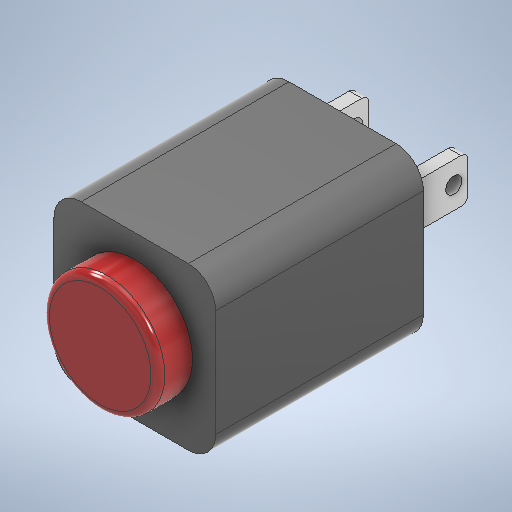
# Autodesk Inventor part: PWR BTN
Saved by Autodesk Inventor 2025 (Build 290162000, 162)
## iProperties
Created: 2025-05-10
Part Number: PWR BTN
Material: Generic
Document SubType Name: Modeling
Designer: thesn
Density: 1 g/cm^3
Appearance: Default
Author: thesn
Autodesk Inventor part; units mm, degrees
ref_plane "YZ Plane" through (0, 0, 0) normal (1, 0, 0) x (0, 1, 0)
ref_plane "XZ Plane" through (0, 0, 0) normal (0, 1, 0) x (-1, 0, 0)
ref_plane "XY Plane" through (0, 0, 0) normal (0, 0, 1) x (1, 0, 0)
sketch "Sketch1" plane through (0, 0, 0) normal (0, 0, 1) x (1, 0, 0)
  line L0 (0, 0) -> (17.78, 0)
  line L1 (17.78, 0) -> (17.78, 17.78)
  line L2 (17.78, 17.78) -> (0, 17.78)
  line L3 (0, 17.78) -> (0, 0)
  dimension "d0" = 17.78
  dimension "d1" = 17.78
  constraints: 8 end point, 2 parallel, 1 horizontal, 1 perpendicular
  measures "d0" distance of L2.end L1.end
  measures "d1" distance of L1.end L0.end
extrude "Extrusion1" add sketch "Sketch1" against normal blind 22.86
fillet "Fillet1" radius 3 4 edges at (17.78, 17.78, -11.43) (0, 17.78, -11.43) (17.78, 0, -11.43) (0, 0, -11.43)
sketch "Sketch2" plane through (0, 0, 0) normal (0, 0, 1) x (1, 0, 0)
  circle A0 centre (8.89, 8.89) radius 6.35
  line L0 (14.78, 17.78) -> (3, 17.78) projected
  line L1 (0, 14.78) -> (0, 3) projected
  point P0 (0, 0)
  point P1 (8.89, 17.78)
  point P2 (0, 8.89)
  dimension "d5" = 0
  dimension "d6" = 0
  dimension "d7" = 12.7
  constraints: 2 midpoint, 1 centre point
  measures "d5" horizontal distance of point (8.89, 17.78) A0.centre
  measures "d6" vertical distance of point (0, 8.89) A0.centre
  measures "d7" diameter of A0
extrude "Extrusion2" add sketch "Sketch2" along normal blind 3.81
fillet "Fillet2" radius 0.762 1 edges at (2.54, 8.89, 3.81)
sketch "Sketch3" plane through (0, 0, -22.86) normal (0, 0, -1) x (-1, 0, 0)
  line L0 (-15.0625, 13.3567) -> (-13.6709, 13.3567)
  line L1 (-13.6709, 13.3567) -> (-13.6709, 8.5084)
  line L2 (-13.6709, 8.5084) -> (-15.0625, 8.5084)
  line L3 (-15.0625, 8.5084) -> (-15.0625, 13.3567)
  line L4 (-4.1566, 13.3567) -> (-2.7649, 13.3567)
  line L5 (-2.7649, 13.3567) -> (-2.7649, 8.5084)
  line L6 (-2.7649, 8.5084) -> (-4.1566, 8.5084)
  line L7 (-4.1566, 8.5084) -> (-4.1566, 13.3567)
  line L8 (-3, 17.78) -> (-14.78, 17.78) projected
  point P0 (0, 0)
  point P1 (-3.4608, 13.3567)
  point P2 (-14.3667, 13.3567)
  point P3 (-8.89, 17.78)
  dimension "d11" = 0
  dimension "d12" = 5.4767
  dimension "d13" = 1.3916
  dimension "d14" = 4.8482
  dimension "d15" = 4.8482
  dimension "d16" = 1.3916
  constraints: 16 end point, 4 parallel, 3 midpoint, 2 horizontal, 2 perpendicular
  measures "d11" vertical distance of point (-3.461, 13.357) point (-14.367, 13.357)
  measures "d12" horizontal distance of point (-8.89, 17.78) point (-14.367, 13.357)
  measures "d13" distance between parallel lines of L1 L3
  measures "d14" distance between parallel lines of L2 L0
  measures "d15" distance between parallel lines of L6 L4
  measures "d16" distance between parallel lines of L7 L5
extrude "Extrusion3" add sketch "Sketch3" along normal blind 7.62
sketch "Sketch4" plane through (2.7649, 8.5084, -22.86) normal (-1, 0, 0) x (0, 0, 1)
  circle A0 centre (-6.0701, 2.4241) radius 0.889
  point P0 (22.86, -8.5084)
  dimension "d19" = 1.778
  constraints: 1 centre point
  measures "d19" diameter of A0
extrude "Extrusion4" cut sketch "Sketch4" against normal blind 25.4
fillet "Fillet3" radius 0.762 4 edges at (14.3667, 13.3567, -30.48) (3.4608, 13.3567, -30.48) (14.3667, 8.5084, -30.48) (3.4608, 8.5084, -30.48)
sketch "Sketch5" plane through (0, 0, -22.86) normal (0, 0, -1) x (-1, 0, 0)
  line L0 (-16.1365, 4.1263) -> (18.4067, 4.1263) construction
  line L1 (18.4067, 4.1263) -> (18.4067, 0.8585) construction
  line L2 (18.4067, 0.8585) -> (-16.1365, 0.8585) construction
  line L3 (-16.1365, 0.8585) -> (-16.1365, 4.1263) construction
  line L4 (-16.1448, 2.7914) -> (-15.7166, 4.0614)
  line L5 (-15.7166, 4.0614) -> (-15.5087, 4.0614)
  line L6 (-15.5087, 4.0614) -> (-15.0806, 2.7914)
  line L7 (-15.0806, 2.7914) -> (-15.2586, 2.7914)
  line L8 (-15.2586, 2.7914) -> (-15.3739, 3.1465)
  line L9 (-15.3739, 3.1465) -> (-15.8586, 3.1465)
  line L10 (-15.8586, 3.1465) -> (-15.9739, 2.7914)
  line L11 (-15.9739, 2.7914) -> (-16.1448, 2.7914)
  line L12 (-15.4202, 3.2906) -> (-15.6168, 3.8885)
  line L13 (-15.6168, 3.8885) -> (-15.8123, 3.2906)
  line L14 (-15.8123, 3.2906) -> (-15.4202, 3.2906)
  line L15 (-14.2398, 2.7914) -> (-14.4003, 2.7914)
  line L16 (-14.4003, 2.7914) -> (-14.4003, 2.8882)
  spline S0 degree 2 poles (-14.4003, 2.8882) (-14.4374, 2.8573) (-14.4919, 2.8161) (-14.5289, 2.7987) knots 0 0 0 1 2 2 2
  spline S1 degree 2 poles (-14.5289, 2.7987) (-14.5629, 2.7822) (-14.636, 2.7647) (-14.6844, 2.7647) knots 0 0 0 1 2 2 2
  spline S2 degree 2 poles (-14.6844, 2.7647) (-14.7626, 2.7647) (-14.8943, 2.8295) (-14.9406, 2.8923) knots 0 0 0 1 2 2 2
  spline S3 degree 2 poles (-14.9406, 2.8923) (-14.9869, 2.9551) (-15.0384, 3.1403) (-15.0384, 3.2608) knots 0 0 0 1 2 2 2
  spline S4 degree 2 poles (-15.0384, 3.2608) (-15.0384, 3.3863) (-14.9736, 3.5695) (-14.9169, 3.6385) knots 0 0 0 1 2 2 2
  spline S5 degree 2 poles (-14.9169, 3.6385) (-14.8645, 3.7002) (-14.7173, 3.7712) (-14.636, 3.7712) knots 0 0 0 1 2 2 2
  spline S6 degree 2 poles (-14.636, 3.7712) (-14.565, 3.7712) (-14.459, 3.7393) (-14.4003, 3.7064) knots 0 0 0 1 2 2 2
  line L17 (-14.4003, 3.7064) -> (-14.4003, 4.1181)
  line L18 (-14.4003, 4.1181) -> (-14.2398, 4.1181)
  line L19 (-14.2398, 4.1181) -> (-14.2398, 2.7914)
  line L20 (-14.4003, 3.023) -> (-14.4003, 3.5736)
  spline S7 degree 2 poles (-14.4003, 3.5736) (-14.46, 3.6024) (-14.5547, 3.6241) (-14.6092, 3.6241) knots 0 0 0 1 2 2 2
  spline S8 degree 2 poles (-14.6092, 3.6241) (-14.7327, 3.6241) (-14.8727, 3.4388) (-14.8727, 3.2638) knots 0 0 0 1 2 2 2
  spline S9 degree 2 poles (-14.8727, 3.2638) (-14.8727, 3.0951) (-14.7657, 2.917) (-14.6473, 2.917) knots 0 0 0 1 2 2 2
  spline S10 degree 2 poles (-14.6473, 2.917) (-14.5845, 2.917) (-14.4569, 2.9746) (-14.4003, 3.023) knots 0 0 0 1 2 2 2
  spline S11 degree 2 poles (-13.4761, 2.8923) (-13.4957, 2.8779) (-13.5615, 2.8264) (-13.5924, 2.811) knots 0 0 0 1 2 2 2
  spline S12 degree 2 poles (-13.5924, 2.811) (-13.6346, 2.7884) (-13.7138, 2.7647) (-13.7859, 2.7647) knots 0 0 0 1 2 2 2
  spline S13 degree 2 poles (-13.7859, 2.7647) (-13.8445, 2.7647) (-13.9506, 2.8089) (-13.9907, 2.8491) knots 0 0 0 1 2 2 2
  spline S14 degree 2 poles (-13.9907, 2.8491) (-14.0288, 2.8882) (-14.0751, 3.0035) (-14.0751, 3.0673) knots 0 0 0 1 2 2 2
  spline S15 degree 2 poles (-14.0751, 3.0673) (-14.0751, 3.1661) (-13.9917, 3.306) (-13.9012, 3.3462) knots 0 0 0 1 2 2 2
  spline S16 degree 2 poles (-13.9012, 3.3462) (-13.8209, 3.3832) (-13.6027, 3.411) (-13.4761, 3.4182) knots 0 0 0 1 2 2 2
  line L21 (-13.4761, 3.4182) -> (-13.4761, 3.4491)
  spline S17 degree 2 poles (-13.4761, 3.4491) (-13.4761, 3.5047) (-13.5101, 3.5736) (-13.5409, 3.5932) knots 0 0 0 1 2 2 2
  spline S18 degree 2 poles (-13.5409, 3.5932) (-13.5718, 3.6127) (-13.6603, 3.6251) (-13.7077, 3.6251) knots 0 0 0 1 2 2 2
  spline S19 degree 2 poles (-13.7077, 3.6251) (-13.7632, 3.6251) (-13.9135, 3.5921) (-13.9886, 3.5602) knots 0 0 0 1 2 2 2
  line L22 (-13.9886, 3.5602) -> (-13.9979, 3.5602)
  line L23 (-13.9979, 3.5602) -> (-13.9979, 3.7239)
  spline S20 degree 2 poles (-13.9979, 3.7239) (-13.9536, 3.7362) (-13.7879, 3.7671) (-13.7066, 3.7671) knots 0 0 0 1 2 2 2
  spline S21 degree 2 poles (-13.7066, 3.7671) (-13.6078, 3.7671) (-13.473, 3.7362) (-13.4195, 3.6961) knots 0 0 0 1 2 2 2
  spline S22 degree 2 poles (-13.4195, 3.6961) (-13.367, 3.657) (-13.3156, 3.5325) (-13.3156, 3.4429) knots 0 0 0 1 2 2 2
  line L24 (-13.3156, 3.4429) -> (-13.3156, 2.7914)
  line L25 (-13.3156, 2.7914) -> (-13.4761, 2.7914)
  line L26 (-13.4761, 2.7914) -> (-13.4761, 2.8923)
  line L27 (-13.4761, 3.0261) -> (-13.4761, 3.2906)
  spline S23 degree 2 poles (-13.4761, 3.2906) (-13.5337, 3.2855) (-13.7077, 3.268) (-13.7622, 3.2515) knots 0 0 0 1 2 2 2
  spline S24 degree 2 poles (-13.7622, 3.2515) (-13.826, 3.2319) (-13.9094, 3.1506) (-13.9094, 3.0786) knots 0 0 0 1 2 2 2
  spline S25 degree 2 poles (-13.9094, 3.0786) (-13.9094, 2.9963) (-13.8168, 2.9129) (-13.7283, 2.9129) knots 0 0 0 1 2 2 2
  spline S26 degree 2 poles (-13.7283, 2.9129) (-13.6531, 2.9129) (-13.5296, 2.9777) (-13.4761, 3.0261) knots 0 0 0 1 2 2 2
  line L28 (-12.589, 3.9637) -> (-12.5972, 3.9637)
  spline S27 degree 2 poles (-12.5972, 3.9637) (-12.6188, 3.9719) (-12.6991, 3.9863) (-12.731, 3.9863) knots 0 0 0 1 2 2 2
  spline S28 degree 2 poles (-12.731, 3.9863) (-12.8318, 3.9863) (-12.9183, 3.8958) (-12.9183, 3.7764) knots 0 0 0 1 2 2 2
  line L29 (-12.9183, 3.7764) -> (-12.9183, 3.7445)
  line L30 (-12.9183, 3.7445) -> (-12.6528, 3.7445)
  line L31 (-12.6528, 3.7445) -> (-12.6528, 3.6117)
  line L32 (-12.6528, 3.6117) -> (-12.9131, 3.6117)
  line L33 (-12.9131, 3.6117) -> (-12.9131, 2.7914)
  line L34 (-12.9131, 2.7914) -> (-13.0737, 2.7914)
  line L35 (-13.0737, 2.7914) -> (-13.0737, 3.6117)
  line L36 (-13.0737, 3.6117) -> (-13.1818, 3.6117)
  line L37 (-13.1818, 3.6117) -> (-13.1818, 3.7445)
  line L38 (-13.1818, 3.7445) -> (-13.0737, 3.7445)
  line L39 (-13.0737, 3.7445) -> (-13.0737, 3.7764)
  spline S29 degree 2 poles (-13.0737, 3.7764) (-13.0737, 3.9472) (-12.908, 4.1263) (-12.7536, 4.1263) knots 0 0 0 1 2 2 2
  spline S30 degree 2 poles (-12.7536, 4.1263) (-12.7094, 4.1263) (-12.6239, 4.117) (-12.589, 4.1108) knots 0 0 0 1 2 2 2
  line L40 (-12.589, 4.1108) -> (-12.589, 3.9637)
  line L41 (-12.0291, 3.5726) -> (-12.0373, 3.5726)
  spline S31 degree 2 poles (-12.0373, 3.5726) (-12.0558, 3.5777) (-12.096, 3.5798) (-12.1238, 3.5798) knots 0 0 0 1 2 2 2
  spline S32 degree 2 poles (-12.1238, 3.5798) (-12.1886, 3.5798) (-12.3162, 3.5232) (-12.3739, 3.4676) knots 0 0 0 1 2 2 2
  line L42 (-12.3739, 3.4676) -> (-12.3739, 2.7914)
  line L43 (-12.3739, 2.7914) -> (-12.5344, 2.7914)
  line L44 (-12.5344, 2.7914) -> (-12.5344, 3.7445)
  line L45 (-12.5344, 3.7445) -> (-12.3739, 3.7445)
  line L46 (-12.3739, 3.7445) -> (-12.3739, 3.6024)
  spline S33 degree 2 poles (-12.3739, 3.6024) (-12.2864, 3.6807) (-12.1557, 3.7445) (-12.0939, 3.7445) knots 0 0 0 1 2 2 2
  spline S34 degree 2 poles (-12.0939, 3.7445) (-12.0692, 3.7445) (-12.0445, 3.7424) (-12.0291, 3.7393) knots 0 0 0 1 2 2 2
  line L47 (-12.0291, 3.7393) -> (-12.0291, 3.5726)
  line L48 (-11.1636, 2.7914) -> (-11.3241, 2.7914)
  line L49 (-11.3241, 2.7914) -> (-11.3241, 2.8964)
  spline S35 degree 2 poles (-11.3241, 2.8964) (-11.3982, 2.8316) (-11.531, 2.7647) (-11.6133, 2.7647) knots 0 0 0 1 2 2 2
  spline S36 degree 2 poles (-11.6133, 2.7647) (-11.6751, 2.7647) (-11.7852, 2.8059) (-11.8253, 2.8501) knots 0 0 0 1 2 2 2
  spline S37 degree 2 poles (-11.8253, 2.8501) (-11.8665, 2.8944) (-11.9118, 3.0292) (-11.9118, 3.1259) knots 0 0 0 1 2 2 2
  line L50 (-11.9118, 3.1259) -> (-11.9118, 3.7445)
  line L51 (-11.9118, 3.7445) -> (-11.7512, 3.7445)
  line L52 (-11.7512, 3.7445) -> (-11.7512, 3.2011)
  spline S38 degree 2 poles (-11.7512, 3.2011) (-11.7512, 3.1249) (-11.7399, 3.0251) (-11.7203, 2.988) knots 0 0 0 1 2 2 2
  spline S39 degree 2 poles (-11.7203, 2.988) (-11.7008, 2.951) (-11.6339, 2.917) (-11.5711, 2.917) knots 0 0 0 1 2 2 2
  spline S40 degree 2 poles (-11.5711, 2.917) (-11.5124, 2.917) (-11.3797, 2.9839) (-11.3241, 3.0323) knots 0 0 0 1 2 2 2
  line L53 (-11.3241, 3.0323) -> (-11.3241, 3.7445)
  line L54 (-11.3241, 3.7445) -> (-11.1636, 3.7445)
  line L55 (-11.1636, 3.7445) -> (-11.1636, 2.7914)
  line L56 (-10.7673, 2.7914) -> (-10.9279, 2.7914)
  line L57 (-10.9279, 2.7914) -> (-10.9279, 3.7445)
  line L58 (-10.9279, 3.7445) -> (-10.7673, 3.7445)
  line L59 (-10.7673, 3.7445) -> (-10.7673, 2.7914)
  line L60 (-10.756, 3.903) -> (-10.9382, 3.903)
  line L61 (-10.9382, 3.903) -> (-10.9382, 4.0697)
  line L62 (-10.9382, 4.0697) -> (-10.756, 4.0697)
  line L63 (-10.756, 4.0697) -> (-10.756, 3.903)
  spline S41 degree 2 poles (-10.2435, 2.7729) (-10.3742, 2.7729) (-10.5213, 2.9222) (-10.5213, 3.0837) knots 0 0 0 1 2 2 2
  line L64 (-10.5213, 3.0837) -> (-10.5213, 3.6117)
  line L65 (-10.5213, 3.6117) -> (-10.6294, 3.6117)
  line L66 (-10.6294, 3.6117) -> (-10.6294, 3.7445)
  line L67 (-10.6294, 3.7445) -> (-10.5213, 3.7445)
  line L68 (-10.5213, 3.7445) -> (-10.5213, 4.0182)
  line L69 (-10.5213, 4.0182) -> (-10.3608, 4.0182)
  line L70 (-10.3608, 4.0182) -> (-10.3608, 3.7445)
  line L71 (-10.3608, 3.7445) -> (-10.0654, 3.7445)
  line L72 (-10.0654, 3.7445) -> (-10.0654, 3.6117)
  line L73 (-10.0654, 3.6117) -> (-10.3608, 3.6117)
  line L74 (-10.3608, 3.6117) -> (-10.3608, 3.1578)
  spline S42 degree 2 poles (-10.3608, 3.1578) (-10.3608, 3.0858) (-10.3557, 3.0065) (-10.3382, 2.9726) knots 0 0 0 1 2 2 2
  spline S43 degree 2 poles (-10.3382, 2.9726) (-10.3237, 2.9427) (-10.2589, 2.9129) (-10.2033, 2.9129) knots 0 0 0 1 2 2 2
  spline S44 degree 2 poles (-10.2033, 2.9129) (-10.1642, 2.9129) (-10.0912, 2.9366) (-10.0747, 2.9438) knots 0 0 0 1 2 2 2
  line L75 (-10.0747, 2.9438) -> (-10.0654, 2.9438)
  line L76 (-10.0654, 2.9438) -> (-10.0654, 2.7997)
  spline S45 degree 2 poles (-10.0654, 2.7997) (-10.1107, 2.7873) (-10.2033, 2.7729) (-10.2435, 2.7729) knots 0 0 0 1 2 2 2
  spline S46 degree 2 poles (-8.5865, 3.6786) (-8.5865, 3.5963) (-8.6452, 3.4481) (-8.6977, 3.3966) knots 0 0 0 1 2 2 2
  spline S47 degree 2 poles (-8.6977, 3.3966) (-8.7635, 3.3318) (-8.9416, 3.2649) (-9.0774, 3.2649) knots 0 0 0 1 2 2 2
  line L77 (-9.0774, 3.2649) -> (-9.2205, 3.2649)
  line L78 (-9.2205, 3.2649) -> (-9.2205, 2.7914)
  line L79 (-9.2205, 2.7914) -> (-9.3893, 2.7914)
  line L80 (-9.3893, 2.7914) -> (-9.3893, 4.0614)
  line L81 (-9.3893, 4.0614) -> (-9.0702, 4.0614)
  spline S48 degree 2 poles (-9.0702, 4.0614) (-8.957, 4.0614) (-8.7985, 4.0244) (-8.7378, 3.9822) knots 0 0 0 1 2 2 2
  spline S49 degree 2 poles (-8.7378, 3.9822) (-8.6668, 3.9338) (-8.5865, 3.7846) (-8.5865, 3.6786) knots 0 0 0 1 2 2 2
  spline S50 degree 2 poles (-8.7625, 3.6735) (-8.7625, 3.7393) (-8.8078, 3.8361) (-8.8541, 3.8669) knots 0 0 0 1 2 2 2
  spline S51 degree 2 poles (-8.8541, 3.8669) (-8.8942, 3.8937) (-9.0013, 3.9153) (-9.0805, 3.9153) knots 0 0 0 1 2 2 2
  line L82 (-9.0805, 3.9153) -> (-9.2205, 3.9153)
  line L83 (-9.2205, 3.9153) -> (-9.2205, 3.409)
  line L84 (-9.2205, 3.409) -> (-9.1052, 3.409)
  spline S52 degree 2 poles (-9.1052, 3.409) (-9.0023, 3.409) (-8.8757, 3.4419) (-8.8345, 3.4851) knots 0 0 0 1 2 2 2
  spline S53 degree 2 poles (-8.8345, 3.4851) (-8.7965, 3.5232) (-8.7625, 3.6127) (-8.7625, 3.6735) knots 0 0 0 1 2 2 2
  line L85 (-7.9834, 2.7914) -> (-8.4754, 2.7914)
  line L86 (-8.4754, 2.7914) -> (-8.4754, 2.9211)
  line L87 (-8.4754, 2.9211) -> (-8.3138, 2.9211)
  line L88 (-8.3138, 2.9211) -> (-8.3138, 3.9318)
  line L89 (-8.3138, 3.9318) -> (-8.4754, 3.9318)
  line L90 (-8.4754, 3.9318) -> (-8.4754, 4.0614)
  line L91 (-8.4754, 4.0614) -> (-7.9834, 4.0614)
  line L92 (-7.9834, 4.0614) -> (-7.9834, 3.9318)
  line L93 (-7.9834, 3.9318) -> (-8.145, 3.9318)
  line L94 (-8.145, 3.9318) -> (-8.145, 2.9211)
  line L95 (-8.145, 2.9211) -> (-7.9834, 2.9211)
  line L96 (-7.9834, 2.9211) -> (-7.9834, 2.7914)
  spline S54 degree 2 poles (-6.7731, 3.4254) (-6.7731, 3.2515) (-6.9141, 2.9716) (-7.0324, 2.8933) knots 0 0 0 1 2 2 2
  spline S55 degree 2 poles (-7.0324, 2.8933) (-7.1292, 2.8326) (-7.3278, 2.7914) (-7.4822, 2.7914) knots 0 0 0 1 2 2 2
  line L97 (-7.4822, 2.7914) -> (-7.7745, 2.7914)
  line L98 (-7.7745, 2.7914) -> (-7.7745, 4.0614)
  line L99 (-7.7745, 4.0614) -> (-7.4853, 4.0614)
  spline S56 degree 2 poles (-7.4853, 4.0614) (-7.3062, 4.0614) (-7.1024, 4.0079) (-7.0304, 3.9606) knots 0 0 0 1 2 2 2
  spline S57 degree 2 poles (-7.0304, 3.9606) (-6.9079, 3.8793) (-6.7731, 3.6107) (-6.7731, 3.4254) knots 0 0 0 1 2 2 2
  spline S58 degree 2 poles (-6.9491, 3.4275) (-6.9491, 3.5736) (-7.0458, 3.7805) (-7.1415, 3.8391) knots 0 0 0 1 2 2 2
  spline S59 degree 2 poles (-7.1415, 3.8391) (-7.2095, 3.8793) (-7.3628, 3.9153) (-7.4771, 3.9153) knots 0 0 0 1 2 2 2
  line L100 (-7.4771, 3.9153) -> (-7.6057, 3.9153)
  line L101 (-7.6057, 3.9153) -> (-7.6057, 2.9376)
  line L102 (-7.6057, 2.9376) -> (-7.4771, 2.9376)
  spline S60 degree 2 poles (-7.4771, 2.9376) (-7.3649, 2.9376) (-7.1951, 2.9736) (-7.1261, 3.022) knots 0 0 0 1 2 2 2
  spline S61 degree 2 poles (-7.1261, 3.022) (-7.0376, 3.0817) (-6.9491, 3.2793) (-6.9491, 3.4275) knots 0 0 0 1 2 2 2
  line L103 (-6.3079, 2.7914) -> (-6.5117, 2.7914)
  line L104 (-6.5117, 2.7914) -> (-6.5117, 3.0343)
  line L105 (-6.5117, 3.0343) -> (-6.3079, 3.0343)
  line L106 (-6.3079, 3.0343) -> (-6.3079, 2.7914)
  line L107 (-6.3079, 3.5016) -> (-6.5117, 3.5016)
  line L108 (-6.5117, 3.5016) -> (-6.5117, 3.7445)
  line L109 (-6.5117, 3.7445) -> (-6.3079, 3.7445)
  line L110 (-6.3079, 3.7445) -> (-6.3079, 3.5016)
  line L111 (-4.7436, 2.7914) -> (-5.3631, 2.7914)
  line L112 (-5.3631, 2.7914) -> (-5.3631, 2.9211)
  line L113 (-5.3631, 2.9211) -> (-5.1326, 2.9211)
  line L114 (-5.1326, 2.9211) -> (-5.1326, 3.7723)
  line L115 (-5.1326, 3.7723) -> (-5.3631, 3.7723)
  line L116 (-5.3631, 3.7723) -> (-5.3631, 3.8885)
  spline S62 degree 2 poles (-5.3631, 3.8885) (-5.2324, 3.8885) (-5.1089, 3.9626) (-5.1007, 4.0656) knots 0 0 0 1 2 2 2
  line L117 (-5.1007, 4.0656) -> (-4.969, 4.0656)
  line L118 (-4.969, 4.0656) -> (-4.969, 2.9211)
  line L119 (-4.969, 2.9211) -> (-4.7436, 2.9211)
  line L120 (-4.7436, 2.9211) -> (-4.7436, 2.7914)
  line L121 (-3.6928, 3.2278) -> (-3.8441, 3.2278)
  line L122 (-3.8441, 3.2278) -> (-3.8441, 2.7914)
  line L123 (-3.8441, 2.7914) -> (-4.0077, 2.7914)
  line L124 (-4.0077, 2.7914) -> (-4.0077, 3.2278)
  line L125 (-4.0077, 3.2278) -> (-4.5686, 3.2278)
  line L126 (-4.5686, 3.2278) -> (-4.5686, 3.4069)
  line L127 (-4.5686, 3.4069) -> (-4.0005, 4.0614)
  line L128 (-4.0005, 4.0614) -> (-3.8441, 4.0614)
  line L129 (-3.8441, 4.0614) -> (-3.8441, 3.3647)
  line L130 (-3.8441, 3.3647) -> (-3.6928, 3.3647)
  line L131 (-3.6928, 3.3647) -> (-3.6928, 3.2278)
  line L132 (-4.0077, 3.3647) -> (-4.0077, 3.8608)
  line L133 (-4.0077, 3.8608) -> (-4.4348, 3.3647)
  line L134 (-4.4348, 3.3647) -> (-4.0077, 3.3647)
  line L135 (-2.7398, 3.2278) -> (-2.8911, 3.2278)
  line L136 (-2.8911, 3.2278) -> (-2.8911, 2.7914)
  line L137 (-2.8911, 2.7914) -> (-3.0547, 2.7914)
  line L138 (-3.0547, 2.7914) -> (-3.0547, 3.2278)
  line L139 (-3.0547, 3.2278) -> (-3.6156, 3.2278)
  line L140 (-3.6156, 3.2278) -> (-3.6156, 3.4069)
  line L141 (-3.6156, 3.4069) -> (-3.0475, 4.0614)
  line L142 (-3.0475, 4.0614) -> (-2.8911, 4.0614)
  line L143 (-2.8911, 4.0614) -> (-2.8911, 3.3647)
  line L144 (-2.8911, 3.3647) -> (-2.7398, 3.3647)
  line L145 (-2.7398, 3.3647) -> (-2.7398, 3.2278)
  line L146 (-3.0547, 3.3647) -> (-3.0547, 3.8608)
  line L147 (-3.0547, 3.8608) -> (-3.4818, 3.3647)
  line L148 (-3.4818, 3.3647) -> (-3.0547, 3.3647)
  line L149 (-1.8207, 2.7914) -> (-2.6039, 2.7914)
  line L150 (-2.6039, 2.7914) -> (-2.6039, 2.9716)
  spline S63 degree 2 poles (-2.6039, 2.9716) (-2.5195, 3.0508) (-2.3693, 3.198) (-2.2972, 3.2772) knots 0 0 0 1 2 2 2
  spline S64 degree 2 poles (-2.2972, 3.2772) (-2.1521, 3.4367) (-2.0461, 3.6282) (-2.0461, 3.7301) knots 0 0 0 1 2 2 2
  spline S65 degree 2 poles (-2.0461, 3.7301) (-2.0461, 3.7836) (-2.079, 3.8638) (-2.1089, 3.8896) knots 0 0 0 1 2 2 2
  spline S66 degree 2 poles (-2.1089, 3.8896) (-2.1387, 3.9153) (-2.2169, 3.941) (-2.2643, 3.941) knots 0 0 0 1 2 2 2
  spline S67 degree 2 poles (-2.2643, 3.941) (-2.3096, 3.941) (-2.4022, 3.9184) (-2.4444, 3.9009) knots 0 0 0 1 2 2 2
  spline S68 degree 2 poles (-2.4444, 3.9009) (-2.4804, 3.8865) (-2.5473, 3.8453) (-2.5679, 3.8309) knots 0 0 0 1 2 2 2
  line L151 (-2.5679, 3.8309) -> (-2.5772, 3.8309)
  line L152 (-2.5772, 3.8309) -> (-2.5772, 4.012)
  spline S69 degree 2 poles (-2.5772, 4.012) (-2.5247, 4.0378) (-2.3363, 4.0882) (-2.2519, 4.0882) knots 0 0 0 1 2 2 2
  spline S70 degree 2 poles (-2.2519, 4.0882) (-2.0739, 4.0882) (-1.8732, 3.8999) (-1.8732, 3.7393) knots 0 0 0 1 2 2 2
  spline S71 degree 2 poles (-1.8732, 3.7393) (-1.8732, 3.6642) (-1.9082, 3.5386) (-1.9391, 3.4851) knots 0 0 0 1 2 2 2
  spline S72 degree 2 poles (-1.9391, 3.4851) (-1.9699, 3.4295) (-2.0595, 3.3204) (-2.1089, 3.268) knots 0 0 0 1 2 2 2
  spline S73 degree 2 poles (-2.1089, 3.268) (-2.1892, 3.1805) (-2.3857, 2.9932) (-2.4444, 2.9386) knots 0 0 0 1 2 2 2
  line L153 (-2.4444, 2.9386) -> (-1.8207, 2.9386)
  line L154 (-1.8207, 2.9386) -> (-1.8207, 2.7914)
  point P0 (0, 0)
  constraints: 2 other
extrude "Extrusion5" cut sketch "Sketch5" against normal blind 0.254
body "Solid1"
